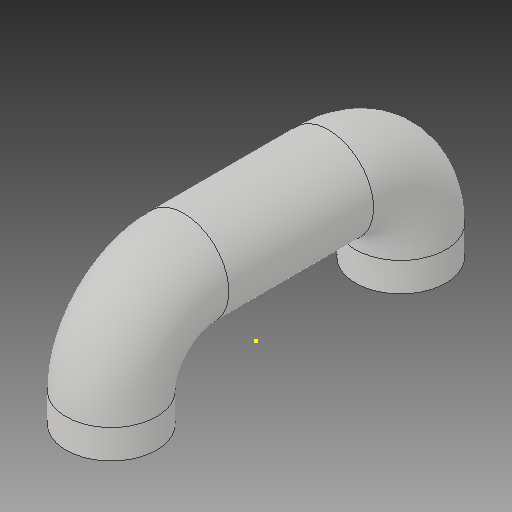
# Autodesk Inventor part: Tube for ball screew
Saved by Autodesk Inventor 2018 (Build 220112000, 112)
## iProperties
Created: 2017-07-25
Part Number: Tube for ball screew
Material: Generic
Document SubType Name: Modeling
Designer: M227562
Density: 1 g/cm^3
Appearance: Default
Author: M227562
Autodesk Inventor part; units mm, degrees
ref_plane "YZ Plane" through (0, 0, 0) normal (1, 0, 0) x (0, 1, 0)
ref_plane "XZ Plane" through (0, 0, 0) normal (0, 1, 0) x (-1, 0, 0)
ref_plane "XY Plane" through (0, 0, 0) normal (0, 0, 1) x (1, 0, 0)
sketch "Sketch1" plane through (0, 0, 0) normal (1, 0, 0) x (0, 1, 0)
  line L0 (0, 0) -> (8.4, 0)
  line L1 (8.4, 0) -> (8.4, 6)
  line L2 (2.4, 12) -> (0, 12)
  arc A0 (8.4, 6) -> (2.4, 12) centre (2.4, 6) ccw
  line L3 (8.4, 0) -> (8.4, -6)
  line L4 (2.4, -12) -> (0, -12)
  arc A1 (2.4, -12) -> (8.4, -6) centre (2.4, -6) ccw
  dimension "d1" = 12
  dimension "d2" = 12
  dimension "d5" = 6
  dimension "d6" = 6
  constraints: 10 end point, 4 point on circle, 4 tangent, 2 centre point, 2 perpendicular, 2 vertical, 1 coincident, 1 horizontal
  measures "d1" distance of L0.start L2.end
  measures "d2" distance of L0.start L4.end
  measures "d5" radius of A0
  measures "d6" radius of A1
sketch "Sketch2" plane through (0, 0, 0) normal (0, 1, 0) x (-1, 0, 0)
  line L0 (0, 0) -> (0, 12)
  circle A0 centre (0, 12) radius 3.75
  dimension "d7" = 12
  dimension "d8" = 7.5
  constraints: 2 end point, 1 centre point, 1 coincident, 1 vertical
  measures "d7" distance of L0.start L0.end
  measures "d8" diameter of A0
sweep "Sweep1" add profiles "Sketch2" path "Sketch1" path curves L2 A0 L1 L3 A1 L4
sketch "Sketch3" plane through (0, 0, -12) normal (0, -1, 0) x (1, 0, 0)
  point P0 (0, 12)
body "Solid1"
